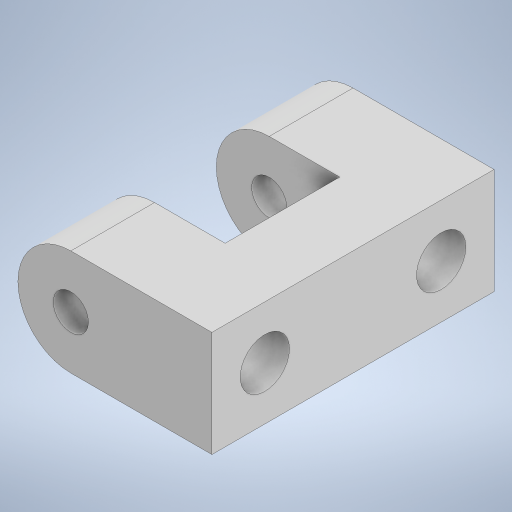
# Autodesk Inventor part: drzak_pritlaku
Saved by Autodesk Inventor 2023 (Build 270158000, 158)
## iProperties
Created: 2023-01-11
Part Number: drzak_pritlaku
Material: Generic
Document SubType Name: Modeling
Designer: zavrel
Density: 1 g/cm^3
Appearance: Default
Author: zavrel
Autodesk Inventor part; units mm, degrees
ref_plane "YZ Plane" through (0, 0, 0) normal (1, 0, 0) x (0, 1, 0)
ref_plane "XZ Plane" through (0, 0, 0) normal (0, 1, 0) x (-1, 0, 0)
ref_plane "XY Plane" through (0, 0, 0) normal (0, 0, 1) x (1, 0, 0)
sketch "Sketch7" plane through (0, 0, 0) normal (0, 1, 0) x (-1, 0, 0)
  line L0 (0, 0) -> (0, -16)
  line L1 (0, -16) -> (11, -16)
  line L2 (11, -16) -> (11, -11.25)
  line L3 (11, -11.25) -> (4, -11.25)
  line L4 (4, -11.25) -> (4, -4.75)
  line L5 (4, -4.75) -> (11, -4.75)
  line L6 (11, -4.75) -> (11, 0)
  line L7 (11, 0) -> (0, 0)
  dimension "d25" = 16
  dimension "d26" = 6.5
  dimension "d27" = 7
  dimension "d28" = 4
  constraints: 16 end point, 6 perpendicular, 2 point on line, 1 collinear, 1 vertical
  measures "d25" distance of L0.start L0.end
  measures "d26" distance between parallel lines of L3 L5
  measures "d27" distance between parallel lines of L6 L4
  measures "d28" distance between parallel lines of L4 L0
extrude "Extrusion7" add sketch "Sketch7" along normal blind 6
sketch "Sketch8" plane through (0, 0, 0) normal (1, 0, 0) x (0, 0, -1)
  line L0 (0, 0) -> (16, 0) projected
  line L1 (16, 0) -> (16, 6) projected
  line L2 (16, 6) -> (0, 6) projected
  line L3 (0, 0) -> (0, 6) projected
  line L4 (4.75, 6) -> (11.25, 6) construction
  line L5 (8, 6) -> (8, 0) construction
  line L6 (11.25, 0) -> (4.75, 0) construction
  line L7 (16, 0) -> (16, 6) construction
  line L8 (16, 3) -> (0, 3) construction
  line L9 (0, 0) -> (0, 6) construction
  circle A0 centre (3, 3) radius 1.4
  circle A1 centre (13, 3) radius 1.4
  dimension "d31" = 2.8
  dimension "d32" = 10
  constraints: 4 end point, 4 midpoint, 2 centre point, 1 point on line, 1 symmetric about line, 1 other
  measures "d31" diameter of A0
  measures "d32" distance of A1.centre A0.centre
extrude "Extrusion8" cut sketch "Sketch8" against normal blind 6 contours A0 | A1
sketch "Sketch9" plane through (-11, 0, 0) normal (0, 0, 1) x (1, 0, 0)
  line L0 (0, 0) -> (11, 0) projected
  line L1 (11, 0) -> (11, 6) projected
  line L2 (11, 6) -> (0, 6) projected
  line L3 (0, 0) -> (0, 6) projected
  line L4 (11, 0) -> (11, 6) construction
  line L5 (11, 3) -> (0, 3) construction
  circle A0 centre (3, 3) radius 1
  dimension "d35" = 2
  dimension "d36" = 3
  constraints: 2 end point, 2 midpoint, 1 centre point, 1 point on line
  measures "d35" diameter of A0
  measures "d36" distance from line of L3 A0.centre
extrude "Extrusion9" cut sketch "Sketch9" against normal through all contours A0
fillet "Fillet2" radius 3 4 edges at (-11, 6, -13.625) (-11, 0, -13.625) (-11, 6, -2.375) (-11, 0, -2.375)
body "Solid2"
